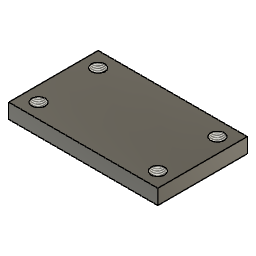
design&manufacturing_simulation (Autodesk Fusion 360 design; units mm, degrees)
Autodesk Fusion 360 part; units mm, degrees
note: some values were not read from the file. Set by a fixed rule: which sketch regions a step uses.
sketch "Sketch1" plane through (0, 0, 0) normal (0, 0, 1) x (1, 0, 0)
  line L0 (-100, 60) -> (100, 60)
  line L1 (100, 60) -> (100, -60)
  line L2 (100, -60) -> (-100, -60)
  line L3 (-100, -60) -> (-100, 60)
  line L4 (-100, 60) -> (100, -60) construction
  line L5 (100, 60) -> (-100, -60) construction
  constraint horizontal L0
  constraint perpendicular L0 L1
  constraint parallel L0 L2
  constraint parallel L1 L3
  constraint coincident L4 origin
  constraint coincident L5 origin
extrude "Extrude1" add sketch "Sketch1" along normal blind 20
sketch "Sketch2" plane through (0, 0, 20) normal (0, 0, 1) x (-1, 0, 0)
  line L0 (100, 60) -> (-100, 60)
  line L1 (-100, 60) -> (-100, -60)
  line L2 (-100, -60) -> (100, -60)
  line L3 (100, -60) -> (100, 60)
  line L4 (80, -40) -> (-80, -40)
  line L5 (-80, -40) -> (-80, 40)
  line L6 (-80, 40) -> (80, 40)
  line L7 (80, 40) -> (80, -40)
  line L8 (80, -40) -> (-80, 40) construction
  line L9 (-80, -40) -> (80, 40) construction
  constraint horizontal L4
  constraint perpendicular L4 L5
  constraint parallel L4 L6
  constraint parallel L5 L7
  constraint coincident L8 origin
  constraint coincident L9 origin
hole "Hole1" at (-80, 40, 20) at (-80, -40, 20) at (80, 40, 20) at (80, -40, 20) direction (0, 0, -1) diameter 18.022 depth 20 tip angle 118
thread "Thread1" "ISO Metric profile 20.0 M20x2 6H"
